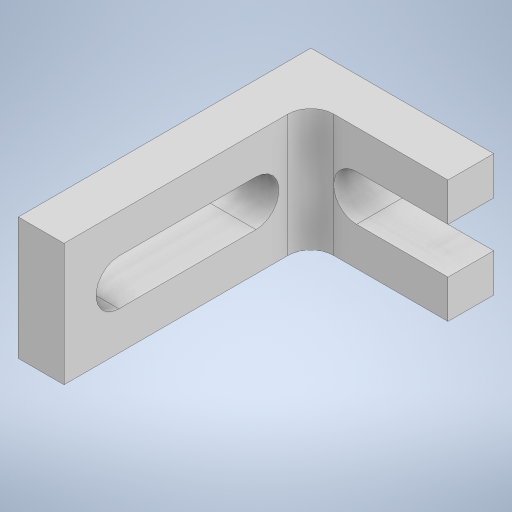
# Autodesk Inventor part: BLKbackplaneBracketMid
Saved by Autodesk Inventor 2023.4 (Build 274418000, 418)
## iProperties
Created: 2024-09-16
Part Number: BLKbackplaneBracketMid
Material: Generic
Document SubType Name: Modeling
Designer: sawtelles
Density: 1 g/cm^3
Appearance: Default
Author: sawtelles
Autodesk Inventor part; units mm, degrees
ref_plane "YZ Plane" through (0, 0, 0) normal (1, 0, 0) x (0, 1, 0)
ref_plane "XZ Plane" through (0, 0, 0) normal (0, 1, 0) x (-1, 0, 0)
ref_plane "XY Plane" through (0, 0, 0) normal (0, 0, 1) x (1, 0, 0)
sketch "Sketch1" plane through (0, 0, 0) normal (0, 0, 1) x (1, 0, 0)
  line L0 (0, 0) -> (50.8, 0)
  line L1 (50.8, 0) -> (50.8, 19.05)
  line L2 (50.8, 19.05) -> (0, 19.05)
  line L3 (0, 19.05) -> (0, 0)
  dimension "d0" = 50.8
  dimension "d1" = 19.05
  constraints: 8 end point, 2 parallel, 1 horizontal, 1 perpendicular
  measures "d0" distance of L2.end L1.end
  measures "d1" distance of L1.end L0.end
extrude "Extrusion1" add sketch "Sketch1" along normal blind 6.35
sketch "Sketch2" plane through (0, 0, 6.35) normal (0, 0, 1) x (1, 0, 0)
  line L0 (0, 19.05) -> (0, 0) projected
  line L1 (50.8, 19.05) -> (0, 19.05) projected
  line L2 (0, 0) -> (6.35, 0)
  line L3 (6.35, 0) -> (6.35, 19.05)
  line L4 (6.35, 19.05) -> (0, 19.05)
  line L5 (0, 19.05) -> (0, 0)
  dimension "d4" = 6.35
  constraints: 8 end point, 2 parallel, 1 horizontal, 1 perpendicular, 1 point on line
  measures "d4" distance of L4.end L3.end
extrude "Extrusion2" add sketch "Sketch2" along normal blind 34.29
sketch "Sketch3" plane through (6.35, 0, 6.35) normal (1, 0, 0) x (0, 0, -1)
  line L0 (-26.67, 9.525) -> (-7.62, 9.525) construction
  line L1 (-26.67, 6.35) -> (-7.62, 6.35)
  line L2 (-7.62, 12.7) -> (-26.67, 12.7)
  arc A0 (-26.67, 12.7) -> (-26.67, 6.35) centre (-26.67, 9.525) ccw
  arc A1 (-7.62, 6.35) -> (-7.62, 12.7) centre (-7.62, 9.525) ccw
  point P0 (6.35, 0)
  point P1 (-17.145, 9.525)
  dimension "d7" = 9.525
  dimension "d8" = 6.35
  constraints: 8 end point, 4 point on circle, 4 tangent, 2 centre point, 1 horizontal, 1 midpoint, 1 parallel
  measures "d7" distance of point (-17.145, 9.525) L0.end
  measures "d8" diameter of A1
extrude "Extrusion3" cut sketch "Sketch3" against normal blind 34.29
sketch "Sketch4" plane through (0, 0, 6.35) normal (0, 0, 1) x (1, 0, 0)
  line L0 (44.45, 9.525) -> (12.7, 9.525) construction
  line L1 (44.45, 12.7) -> (12.7, 12.7)
  line L2 (12.7, 6.35) -> (44.45, 6.35)
  arc A0 (44.45, 6.35) -> (44.45, 12.7) centre (44.45, 9.525) ccw
  arc A1 (12.7, 12.7) -> (12.7, 6.35) centre (12.7, 9.525) ccw
  point P0 (0, 0)
  point P1 (28.575, 9.525)
  dimension "d11" = 15.875
  dimension "d12" = 6.35
  constraints: 8 end point, 4 point on circle, 4 tangent, 2 centre point, 1 horizontal, 1 midpoint, 1 parallel
  measures "d11" distance of point (28.575, 9.525) L0.end
  measures "d12" diameter of A1
extrude "Extrusion4" cut sketch "Sketch4" against normal blind 34.29
fillet "Fillet1" radius 3.175 1 edges at (6.35, 9.525, 6.35)
sketch "Sketch5" plane through (50.8, 0, 0) normal (1, 0, 0) x (0, 0, -1)
  line L0 (0, 19.05) -> (-40.64, 19.05) projected
  line L1 (0, 19.05) -> (-41.8279, 19.05)
  line L2 (-41.8279, 19.05) -> (-41.8279, 18.0326)
  line L3 (-41.8279, 18.0326) -> (0, 18.0326)
  line L4 (0, 18.0326) -> (0, 19.05)
  line L5 (0, 19.05) -> (0, 0) projected
  line L6 (-40.64, 0) -> (-40.64, 19.05) projected
  line L7 (0, 0) -> (-40.64, 0)
  line L8 (-40.64, 0) -> (-40.64, 1.0192)
  line L9 (-40.64, 1.0192) -> (0, 1.0192)
  line L10 (0, 1.0192) -> (0, 0)
  constraints: 16 end point, 4 parallel, 2 horizontal, 2 perpendicular, 1 point on line
extrude "Extrusion5" cut sketch "Sketch5" against normal through all contours L4 L3 L6 L0 | L6 L3 L2 L1 | L5 L7 L6 L9
sketch "Sketch6" plane through (0, 0, 0) normal (0, 0, -1) x (-1, 0, 0)
  line L0 (-50.8, 18.0326) -> (-9.525, 18.0326) projected
  line L1 (-25.4, 18.0326) -> (-61.3669, 18.0326)
  line L2 (-61.3669, 18.0326) -> (-61.3669, -3.7914)
  line L3 (-61.3669, -3.7914) -> (-25.4, -3.7914)
  line L4 (-25.4, -3.7914) -> (-25.4, 18.0326)
  point P0 (0, 0)
  constraints: 8 end point, 2 parallel, 1 horizontal, 1 perpendicular, 1 point on line
extrude "Extrusion6" cut sketch "Sketch6" against normal through all
body "Solid1"
